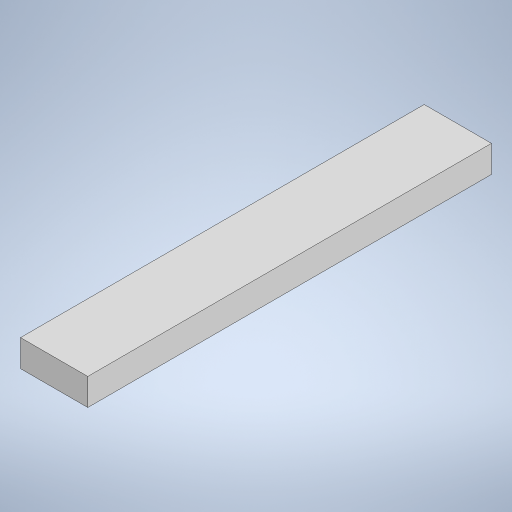
# Autodesk Inventor part: ochrana li-ion baterie
Saved by Autodesk Inventor 2023 (Build 270158000, 158)
## iProperties
Created: 2023-01-20
Part Number: ochrana li-ion baterie
Material: Všeobecné
Document SubType Name: Modeling
Designer: Kuba
Mass: 0.5184 g
Surface Area: 6.336 cm^2
Volume: 0.5184 cm^3
Density: 1 g/cm^3
Appearance: Výchozí
Author: Kuba
Autodesk Inventor part; units mm, degrees
ref_plane "YZ Plane" through (0, 0, 0) normal (1, 0, 0) x (0, 1, 0)
ref_plane "XZ Plane" through (0, 0, 0) normal (0, 1, 0) x (-1, 0, 0)
ref_plane "XY Plane" through (0, 0, 0) normal (0, 0, 1) x (1, 0, 0)
sketch "Náčrt1" plane through (0, 0, 0) normal (0, 0, 1) x (1, 0, 0)
  point P0 (0, 0)
sketch "Náčrt2" plane through (0, 0, 0) normal (0, 1, 0) x (-1, 0, 0)
  line L0 (0, 0) -> (-3, 0)
  line L1 (-3, 0) -> (-3, 18) construction
  line L2 (-3, 18) -> (0, 18) construction
  line L3 (0, 18) -> (0, 0) construction
  line L4 (-3, 18) -> (3, 18)
  line L5 (3, 18) -> (3, -18)
  line L6 (3, -18) -> (-3, -18)
  line L7 (-3, -18) -> (-3, 18)
  dimension "d0" = 3
  dimension "d1" = 18
  dimension "d2" = 6
  dimension "d3" = 36
  constraints: 16 end point, 4 parallel, 2 horizontal, 2 perpendicular
  measures "d0" distance of L1.end L2.end
  measures "d1" distance of L0.end L1.end
  measures "d2" distance of L5.end L6.end
  measures "d3" distance of L4.end L5.end
extrude "Vysunutí1" add sketch "Náčrt2" along normal blind 2.4
